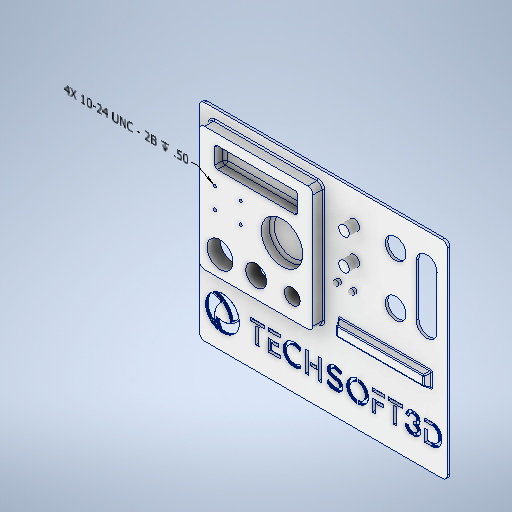
# Autodesk Inventor part: 20250213001
Saved by Autodesk Inventor 2025 (Build 290162000, 162)
## iProperties
Created: 2025-02-13
Part Number: 20250213001
Material: Aluminum 6061
Document SubType Name: Modeling
Designer: beau.trifiro
Density: 2.7 g/cm^3
Appearance: Aluminum - Flat
Description: Sample part
Mass: 1145.53 g
Surface Area: 1662.07 cm^2
Volume: 424.269 cm^3
Company: Tech Soft 3D
Author: beau.trifiro
Title: Sample Part
Revision Number: 0
Autodesk Inventor part; units mm, degrees
(part 1 of 2)
ref_plane "YZ Plane" through (0, 0, 0) normal (1, 0, 0) x (0, 1, 0)
ref_plane "XZ Plane" through (0, 0, 0) normal (0, 1, 0) x (-1, 0, 0)
ref_plane "XY Plane" through (0, 0, 0) normal (0, 0, 1) x (1, 0, 0)
sketch "Sketch1" plane through (0, 0, 0) normal (0, 0, 1) x (1, 0, 0)
  line L0 (-152.4, -127) -> (152.4, -127)
  line L1 (152.4, -127) -> (152.4, 127)
  line L2 (152.4, 127) -> (-152.4, 127)
  line L3 (-152.4, 127) -> (-152.4, -127)
  line L4 (-152.4, -127) -> (152.4, 127) construction
  line L5 (152.4, -127) -> (-152.4, 127) construction
  point P0 (0, 0)
  dimension "d0" = 304.8
  dimension "d1" = 254
  constraints: 12 end point, 2 midpoint, 2 parallel, 1 horizontal, 1 perpendicular
  measures "d0" distance of L1.end L2.end
  measures "d1" distance of L0.end L1.end
extrude "Extrusion1" add sketch "Sketch1" along normal blind 3.175
sketch "Sketch2" plane through (0, 0, 3.175) normal (0, 0, 1) x (1, 0, 0)
  line L0 (-139.7, 114.3) -> (0, 114.3)
  line L1 (0, 114.3) -> (0, -38.1)
  line L2 (0, -38.1) -> (-139.7, -38.1)
  line L3 (-139.7, -38.1) -> (-139.7, 114.3)
  line L4 (152.4, 127) -> (-152.4, 127) projected
  line L5 (-152.4, 127) -> (-152.4, -127) projected
  line L6 (-152.4, -127) -> (152.4, -127) projected
  point P0 (0, 0)
  dimension "d4" = 12.7
  dimension "d5" = 12.7
  dimension "d39" = 152.4
  constraints: 8 end point, 2 parallel, 1 horizontal, 1 perpendicular, 1 vertical alignment
  measures "d4" distance between parallel lines of L4 L0
  measures "d5" distance between parallel lines of L5 L3
  measures "d39" distance of L2.end L0.start
extrude "Extrusion2" add sketch "Sketch2" along normal blind 12.7
sketch "Sketch3" plane through (0, 0, 15.875) normal (0, 0, 1) x (1, 0, 0)
  line L0 (-120.65, 101.6) -> (-19.05, 101.6)
  line L1 (-19.05, 101.6) -> (-19.05, 76.2)
  line L2 (-19.05, 76.2) -> (-120.65, 76.2)
  line L3 (-120.65, 76.2) -> (-120.65, 101.6)
  circle A0 centre (-114.3, -12.7) radius 15.875
  circle A1 centre (-38.1, 38.1) radius 25.4
  circle A2 centre (-25.4, -12.7) radius 9.525
  circle A3 centre (-69.85, -12.7) radius 12.7
  line L4 (-139.7, 114.3) -> (-139.7, -38.1) projected
  line L5 (0, 114.3) -> (-139.7, 114.3) projected
  line L6 (0, -38.1) -> (0, 114.3) projected
  line L7 (-139.7, -38.1) -> (0, -38.1) projected
  line L8 (-120.65, 57.15) -> (-88.9, 57.15) construction
  line L9 (-88.9, 57.15) -> (-88.9, 31.75) construction
  line L10 (-88.9, 31.75) -> (-120.65, 31.75) construction
  line L11 (-120.65, 31.75) -> (-120.65, 57.15) construction
  point P0 (0, 0)
  point P1 (0, 38.1)
  point P2 (0, 38.1)
  dimension "d9" = 19.05
  dimension "d10" = 12.7
  dimension "d11" = 19.05
  dimension "d12" = 25.4
  dimension "d13" = 50.8
  dimension "d14" = 38.1
  dimension "d16" = 31.75
  dimension "d17" = 19.05
  dimension "d19" = 25.4
  dimension "d21" = 25.4
  dimension "d22" = 25.4
  dimension "d23" = 50.8
  dimension "d40" = 44.45
  dimension "d41" = 38.1
  dimension "d42" = 25.4
  dimension "d43" = 31.75
  dimension "d44" = 19.05
  dimension "d45" = 19.05
  constraints: 16 end point, 4 centre point, 4 parallel, 3 horizontal alignment, 2 horizontal, 2 midpoint, 2 perpendicular
  measures "d9" distance between parallel lines of L4 L3
  measures "d10" distance between parallel lines of L5 L0
  measures "d11" distance between parallel lines of L6 L1
  measures "d12" distance between parallel lines of L0 L2
  measures "d13" diameter of A1
  measures "d14" distance from line of L6 A1.centre
  measures "d16" diameter of A0
  measures "d17" diameter of A2
  measures "d19" diameter of A3
  measures "d21" distance from line of L4 A0.centre
  measures "d22" distance from line of L6 A2.centre
  measures "d23" vertical distance of point (0, 38.1) A2.centre
  measures "d40" distance of A2.centre A3.centre
  measures "d42" distance of L8.end L9.end
  measures "d43" distance of L9.end L10.end
  measures "d44" distance between parallel lines of L4 L11
  measures "d45" distance between parallel lines of L2 L8
extrude "Extrusion3" cut sketch "Sketch3" against normal blind 12.7 contours L0 L1 L2 L3
extrude "Extrusion4" cut sketch "Sketch3" against normal blind 12.7 contours A1
extrude "Extrusion5" cut sketch "Sketch3" against normal through all contours A0 | A2 | A3
sketch "Sketch4" plane through (0, 0, 3.175) normal (0, 0, 1) x (1, 0, 0)
  line L0 (127, 88.9) -> (127, 25.4) construction
  line L1 (114.3, 88.9) -> (114.3, 25.4)
  line L2 (139.7, 25.4) -> (139.7, 88.9)
  arc A0 (139.7, 88.9) -> (114.3, 88.9) centre (127, 88.9) ccw
  arc A1 (114.3, 25.4) -> (139.7, 25.4) centre (127, 25.4) ccw
  circle A2 centre (88.9, 88.9) radius 12.7
  circle A3 centre (88.9, 25.4) radius 12.7
  line L3 (152.4, 127) -> (-152.4, 127) projected
  line L4 (152.4, -127) -> (152.4, 127) projected
  circle A4 centre (38.1, 88.9) radius 6.35
  circle A5 centre (38.1, 50.8) radius 6.35
  circle A6 centre (38.1, 19.05) radius 3.175
  line L5 (0, -38.1) -> (0, 114.3) projected
  circle A7 centre (19.05, 19.05) radius 3.175
  line L6 (19.05, -19.05) -> (133.35, -19.05)
  line L7 (133.35, -19.05) -> (133.35, -38.1)
  line L8 (133.35, -38.1) -> (19.05, -38.1)
  line L9 (19.05, -38.1) -> (19.05, -19.05)
  line L10 (-152.4, -127) -> (152.4, -127) projected
  point P0 (0, 0)
  point P1 (127, 57.15)
  point P2 (127, 101.6)
  point P3 (139.7, 57.15)
  point P4 (114.3, 57.15)
  dimension "d55" = 25.4
  dimension "d56" = 25.4
  dimension "d57" = 63.5
  dimension "d58" = 25.4
  dimension "d59" = 25.4
  dimension "d60" = 12.7
  dimension "d61" = 12.7
  dimension "d62" = 12.7
  dimension "d63" = 38.1
  dimension "d64" = 38.1
  dimension "d65" = 6.35
  dimension "d66" = 6.35
  dimension "d67" = 19.05
  dimension "d68" = 19.05
  dimension "d70" = 38.1
  dimension "d71" = 38.1
  dimension "d72" = 107.95
  dimension "d77" = 114.3
  dimension "d78" = 19.05
  dimension "d79" = 88.9
  dimension "d80" = 19.05
  constraints: 16 end point, 8 centre point, 5 point on circle, 4 tangent, 3 horizontal alignment, 3 midpoint, 3 parallel, 3 vertical alignment, 1 horizontal, 1 perpendicular, 1 vertical
  measures "d55" distance from line of L3 point (127, 101.6)
  measures "d56" distance of point (139.7, 57.15) point (114.3, 57.15)
  measures "d57" distance of L0.start L0.end
  measures "d58" diameter of A3
  measures "d59" diameter of A2
  measures "d60" distance between parallel lines of L4 L2
  measures "d61" diameter of A4
  measures "d62" diameter of A5
  measures "d63" distance of A5.centre A4.centre
  measures "d64" distance from line of L5 A4.centre
  measures "d65" diameter of A6
  measures "d66" diameter of A7
  measures "d67" distance of A6.centre A7.centre
  measures "d68" distance from line of L5 A7.centre
  measures "d70" distance from line of L0 A3.centre
  measures "d71" distance from line of L3 A4.centre
  measures "d72" distance from line of L3 A6.centre
  measures "d77" distance of L6.start L6.end
  measures "d78" distance between parallel lines of L4 L7
  measures "d79" distance between parallel lines of L10 L8
  measures "d80" distance of L6.end L7.end
extrude "Extrusion6" cut sketch "Sketch4" against normal through all contours A0 L2 A1 L1 | A2 | A3
hole "Hole1" at (-120.65, 57.15, 15.875) at (-88.9, 57.15, 15.875) at (-88.9, 31.75, 15.875) at (-120.65, 31.75, 15.875) direction (0, 0, -1) diameter 3.683 end through all thread size "10-24 UNC" class "2B" standard "ANSI Unified Screw Threads"
extrude "Extrusion8" add sketch "Sketch4" along normal blind 12.7 contours A4 | A5
extrude "Extrusion9" add sketch "Sketch4" along normal blind 6.35 contours A6 | A7
extrude "Extrusion10" add sketch "Sketch4" along normal blind 6.35 draft -30 contours L6 L7 L8 L9
sketch "Sketch5" plane through (0, 0, 3.175) normal (0, 0, 1) x (1, 0, 0)
  line L0 (-89.5982, -73.346) -> (-72.309, -73.346)
  line L1 (-72.309, -73.346) -> (-72.309, -76.9851)
  line L2 (-72.309, -76.9851) -> (-89.5982, -76.9851)
  line L3 (-89.5982, -76.9851) -> (-89.5982, -73.346)
  line L4 (-82.806, -99.2807) -> (-82.806, -79.0998)
  line L5 (-82.806, -79.0998) -> (-79.1012, -79.0998)
  line L6 (-79.1012, -79.0998) -> (-79.1012, -99.2813)
  line L7 (-79.1012, -99.2813) -> (-82.806, -99.2813)
  line L8 (-82.806, -99.2813) -> (-82.806, -99.2807)
  line L9 (-29.191, -93.0667) -> (-27.6081, -96.5408)
  line L10 (-27.6081, -96.5408) -> (-28.0244, -96.9058)
  line L11 (-28.0244, -96.9058) -> (-28.4615, -97.248)
  line L12 (-28.4615, -97.248) -> (-28.9174, -97.5673)
  line L13 (-28.9174, -97.5673) -> (-29.3903, -97.8637)
  line L14 (-29.3903, -97.8637) -> (-29.8784, -98.1371)
  line L15 (-29.8784, -98.1371) -> (-30.3797, -98.3872)
  line L16 (-30.3797, -98.3872) -> (-30.8924, -98.6141)
  line L17 (-30.8924, -98.6141) -> (-31.4147, -98.8175)
  line L18 (-31.4147, -98.8175) -> (-31.9447, -98.9974)
  line L19 (-31.9447, -98.9974) -> (-32.4805, -99.1537)
  line L20 (-32.4805, -99.1537) -> (-33.0202, -99.2863)
  line L21 (-33.0202, -99.2863) -> (-33.562, -99.395)
  line L22 (-33.562, -99.395) -> (-34.104, -99.4797)
  line L23 (-34.104, -99.4797) -> (-34.6444, -99.5404)
  line L24 (-34.6444, -99.5404) -> (-35.1813, -99.5769)
  line L25 (-35.1813, -99.5769) -> (-35.7128, -99.5891)
  line L26 (-35.7128, -99.5891) -> (-36.4069, -99.5718)
  line L27 (-36.4069, -99.5718) -> (-37.092, -99.5205)
  line L28 (-37.092, -99.5205) -> (-37.7672, -99.4361)
  line L29 (-37.7672, -99.4361) -> (-38.4318, -99.3194)
  line L30 (-38.4318, -99.3194) -> (-39.0848, -99.1712)
  line L31 (-39.0848, -99.1712) -> (-39.7253, -98.9923)
  line L32 (-39.7253, -98.9923) -> (-40.3526, -98.7836)
  line L33 (-40.3526, -98.7836) -> (-40.9657, -98.5459)
  line L34 (-40.9657, -98.5459) -> (-41.5639, -98.2801)
  line L35 (-41.5639, -98.2801) -> (-42.1462, -97.9869)
  line L36 (-42.1462, -97.9869) -> (-42.7119, -97.6673)
  line L37 (-42.7119, -97.6673) -> (-43.26, -97.322)
  line L38 (-43.26, -97.322) -> (-43.7896, -96.9519)
  line L39 (-43.7896, -96.9519) -> (-44.3001, -96.5578)
  line L40 (-44.3001, -96.5578) -> (-44.7904, -96.1405)
  line L41 (-44.7904, -96.1405) -> (-45.2597, -95.701)
  line L42 (-45.2597, -95.701) -> (-45.7072, -95.2399)
  line L43 (-45.7072, -95.2399) -> (-46.1321, -94.7582)
  line L44 (-46.1321, -94.7582) -> (-46.5334, -94.2567)
  line L45 (-46.5334, -94.2567) -> (-46.9103, -93.7362)
  line L46 (-46.9103, -93.7362) -> (-47.262, -93.1975)
  line L47 (-47.262, -93.1975) -> (-47.5876, -92.6416)
  line L48 (-47.5876, -92.6416) -> (-47.8862, -92.0691)
  line L49 (-47.8862, -92.0691) -> (-48.1571, -91.481)
  line L50 (-48.1571, -91.481) -> (-48.3992, -90.8781)
  line L51 (-48.3992, -90.8781) -> (-48.6119, -90.2613)
  line L52 (-48.6119, -90.2613) -> (-48.7942, -89.6312)
  line L53 (-48.7942, -89.6312) -> (-48.9452, -88.9889)
  line L54 (-48.9452, -88.9889) -> (-49.0642, -88.335)
  line L55 (-49.0642, -88.335) -> (-49.1503, -87.6706)
  line L56 (-49.1503, -87.6706) -> (-49.2025, -86.9963)
  line L57 (-49.2025, -86.9963) -> (-49.2201, -86.313)
  line L58 (-49.2201, -86.313) -> (-49.2025, -85.6298)
  line L59 (-49.2025, -85.6298) -> (-49.1503, -84.9555)
  line L60 (-49.1503, -84.9555) -> (-49.0642, -84.291)
  line L61 (-49.0642, -84.291) -> (-48.9452, -83.6371)
  line L62 (-48.9452, -83.6371) -> (-48.7941, -82.9948)
  line L63 (-48.7941, -82.9948) -> (-48.6118, -82.3647)
  line L64 (-48.6118, -82.3647) -> (-48.3992, -81.7478)
  line L65 (-48.3992, -81.7478) -> (-48.157, -81.1449)
  line L66 (-48.157, -81.1449) -> (-47.8861, -80.5568)
  line L67 (-47.8861, -80.5568) -> (-47.5875, -79.9843)
  line L68 (-47.5875, -79.9843) -> (-47.2619, -79.4283)
  line L69 (-47.2619, -79.4283) -> (-46.9102, -78.8897)
  line L70 (-46.9102, -78.8897) -> (-46.5332, -78.3691)
  line L71 (-46.5332, -78.3691) -> (-46.1319, -77.8676)
  line L72 (-46.1319, -77.8676) -> (-45.707, -77.3859)
  line L73 (-45.707, -77.3859) -> (-45.2595, -76.9248)
  line L74 (-45.2595, -76.9248) -> (-44.7901, -76.4852)
  line L75 (-44.7901, -76.4852) -> (-44.2998, -76.0679)
  line L76 (-44.2998, -76.0679) -> (-43.7894, -75.6738)
  line L77 (-43.7894, -75.6738) -> (-43.2597, -75.3037)
  line L78 (-43.2597, -75.3037) -> (-42.7116, -74.9583)
  line L79 (-42.7116, -74.9583) -> (-42.146, -74.6387)
  line L80 (-42.146, -74.6387) -> (-41.5636, -74.3455)
  line L81 (-41.5636, -74.3455) -> (-40.9655, -74.0796)
  line L82 (-40.9655, -74.0796) -> (-40.3523, -73.8419)
  line L83 (-40.3523, -73.8419) -> (-39.7251, -73.6332)
  line L84 (-39.7251, -73.6332) -> (-39.0846, -73.4543)
  line L85 (-39.0846, -73.4543) -> (-38.4316, -73.3061)
  line L86 (-38.4316, -73.3061) -> (-37.7671, -73.1893)
  line L87 (-37.7671, -73.1893) -> (-37.0919, -73.1049)
  line L88 (-37.0919, -73.1049) -> (-36.4068, -73.0536)
  line L89 (-36.4068, -73.0536) -> (-35.7128, -73.0364)
  line L90 (-35.7128, -73.0364) -> (-35.1812, -73.0481)
  line L91 (-35.1812, -73.0481) -> (-34.6442, -73.0834)
  line L92 (-34.6442, -73.0834) -> (-34.1038, -73.1422)
  line L93 (-34.1038, -73.1422) -> (-33.5617, -73.2245)
  line L94 (-33.5617, -73.2245) -> (-33.0198, -73.3303)
  line L95 (-33.0198, -73.3303) -> (-32.48, -73.4597)
  line L96 (-32.48, -73.4597) -> (-31.9442, -73.6126)
  line L97 (-31.9442, -73.6126) -> (-31.4143, -73.7889)
  line L98 (-31.4143, -73.7889) -> (-30.892, -73.9889)
  line L99 (-30.892, -73.9889) -> (-30.3793, -74.2123)
  line L100 (-30.3793, -74.2123) -> (-29.878, -74.4592)
  line L101 (-29.878, -74.4592) -> (-29.39, -74.7297)
  line L102 (-29.39, -74.7297) -> (-28.9171, -75.0237)
  line L103 (-28.9171, -75.0237) -> (-28.4613, -75.3412)
  line L104 (-28.4613, -75.3412) -> (-28.0243, -75.6822)
  line L105 (-28.0243, -75.6822) -> (-27.6081, -76.0467)
  line L106 (-27.6081, -76.0467) -> (-29.191, -79.5196)
  line L107 (-29.191, -79.5196) -> (-29.5272, -79.1895)
  line L108 (-29.5272, -79.1895) -> (-29.8707, -78.8795)
  line L109 (-29.8707, -78.8795) -> (-30.2223, -78.5898)
  line L110 (-30.2223, -78.5898) -> (-30.5829, -78.3204)
  line L111 (-30.5829, -78.3204) -> (-30.9535, -78.0716)
  line L112 (-30.9535, -78.0716) -> (-31.335, -77.8435)
  line L113 (-31.335, -77.8435) -> (-31.7281, -77.6364)
  line L114 (-31.7281, -77.6364) -> (-32.134, -77.4503)
  line L115 (-32.134, -77.4503) -> (-32.5533, -77.2855)
  line L116 (-32.5533, -77.2855) -> (-32.9872, -77.1421)
  line L117 (-32.9872, -77.1421) -> (-33.4364, -77.0203)
  line L118 (-33.4364, -77.0203) -> (-33.9019, -76.9203)
  line L119 (-33.9019, -76.9203) -> (-34.3846, -76.8422)
  line L120 (-34.3846, -76.8422) -> (-34.8853, -76.7862)
  line L121 (-34.8853, -76.7862) -> (-35.4051, -76.7524)
  line L122 (-35.4051, -76.7524) -> (-35.9447, -76.7412)
  line L123 (-35.9447, -76.7412) -> (-36.4374, -76.7536)
  line L124 (-36.4374, -76.7536) -> (-36.9235, -76.7906)
  line L125 (-36.9235, -76.7906) -> (-37.4027, -76.8514)
  line L126 (-37.4027, -76.8514) -> (-37.8741, -76.9356)
  line L127 (-37.8741, -76.9356) -> (-38.3373, -77.0424)
  line L128 (-38.3373, -77.0424) -> (-38.7915, -77.1714)
  line L129 (-38.7915, -77.1714) -> (-39.2363, -77.3218)
  line L130 (-39.2363, -77.3218) -> (-39.671, -77.4932)
  line L131 (-39.671, -77.4932) -> (-40.095, -77.6848)
  line L132 (-40.095, -77.6848) -> (-40.5077, -77.8962)
  line L133 (-40.5077, -77.8962) -> (-40.9086, -78.1266)
  line L134 (-40.9086, -78.1266) -> (-41.2969, -78.3755)
  line L135 (-41.2969, -78.3755) -> (-41.6722, -78.6423)
  line L136 (-41.6722, -78.6423) -> (-42.0338, -78.9264)
  line L137 (-42.0338, -78.9264) -> (-42.3811, -79.2273)
  line L138 (-42.3811, -79.2273) -> (-42.7135, -79.5441)
  line L139 (-42.7135, -79.5441) -> (-43.0304, -79.8765)
  line L140 (-43.0304, -79.8765) -> (-43.3312, -80.2238)
  line L141 (-43.3312, -80.2238) -> (-43.6153, -80.5854)
  line L142 (-43.6153, -80.5854) -> (-43.8821, -80.9606)
  line L143 (-43.8821, -80.9606) -> (-44.1311, -81.3489)
  line L144 (-44.1311, -81.3489) -> (-44.3615, -81.7497)
  line L145 (-44.3615, -81.7497) -> (-44.5729, -82.1624)
  line L146 (-44.5729, -82.1624) -> (-44.7645, -82.5864)
  line L147 (-44.7645, -82.5864) -> (-44.9359, -83.0211)
  line L148 (-44.9359, -83.0211) -> (-45.0863, -83.4658)
  line L149 (-45.0863, -83.4658) -> (-45.2153, -83.9201)
  line L150 (-45.2153, -83.9201) -> (-45.3221, -84.3832)
  line L151 (-45.3221, -84.3832) -> (-45.4063, -84.8546)
  line L152 (-45.4063, -84.8546) -> (-45.4671, -85.3336)
  line L153 (-45.4671, -85.3336) -> (-45.5041, -85.8198)
  line L154 (-45.5041, -85.8198) -> (-45.5165, -86.3124)
  line L155 (-45.5165, -86.3124) -> (-45.5041, -86.805)
  line L156 (-45.5041, -86.805) -> (-45.4671, -87.2912)
  line L157 (-45.4671, -87.2912) -> (-45.4063, -87.7703)
  line L158 (-45.4063, -87.7703) -> (-45.3221, -88.2417)
  line L159 (-45.3221, -88.2417) -> (-45.2153, -88.7048)
  line L160 (-45.2153, -88.7048) -> (-45.0863, -89.159)
  line L161 (-45.0863, -89.159) -> (-44.9359, -89.6038)
  line L162 (-44.9359, -89.6038) -> (-44.7645, -90.0385)
  line L163 (-44.7645, -90.0385) -> (-44.5729, -90.4625)
  line L164 (-44.5729, -90.4625) -> (-44.3615, -90.8752)
  line L165 (-44.3615, -90.8752) -> (-44.1311, -91.2761)
  line L166 (-44.1311, -91.2761) -> (-43.8821, -91.6644)
  line L167 (-43.8821, -91.6644) -> (-43.6153, -92.0397)
  line L168 (-43.6153, -92.0397) -> (-43.3312, -92.4013)
  line L169 (-43.3312, -92.4013) -> (-43.0304, -92.7486)
  line L170 (-43.0304, -92.7486) -> (-42.7135, -93.081)
  line L171 (-42.7135, -93.081) -> (-42.3811, -93.3979)
  line L172 (-42.3811, -93.3979) -> (-42.0338, -93.6987)
  line L173 (-42.0338, -93.6987) -> (-41.6722, -93.9829)
  line L174 (-41.6722, -93.9829) -> (-41.2969, -94.2497)
  line L175 (-41.2969, -94.2497) -> (-40.9086, -94.4987)
  line L176 (-40.9086, -94.4987) -> (-40.5077, -94.7291)
  line L177 (-40.5077, -94.7291) -> (-40.095, -94.9405)
  line L178 (-40.095, -94.9405) -> (-39.671, -95.1322)
  line L179 (-39.671, -95.1322) -> (-39.2363, -95.3035)
  line L180 (-39.2363, -95.3035) -> (-38.7915, -95.454)
  line L181 (-38.7915, -95.454) -> (-38.3373, -95.583)
  line L182 (-38.3373, -95.583) -> (-37.8741, -95.6898)
  line L183 (-37.8741, -95.6898) -> (-37.4027, -95.774)
  line L184 (-37.4027, -95.774) -> (-36.9235, -95.8349)
  line L185 (-36.9235, -95.8349) -> (-36.4374, -95.8718)
  line L186 (-36.4374, -95.8718) -> (-35.9447, -95.8843)
  line L187 (-35.9447, -95.8843) -> (-35.4051, -95.873)
  line L188 (-35.4051, -95.873) -> (-34.8853, -95.8392)
  line L189 (-34.8853, -95.8392) -> (-34.3846, -95.783)
  line L190 (-34.3846, -95.783) -> (-33.9019, -95.7046)
  line L191 (-33.9019, -95.7046) -> (-33.4364, -95.6039)
  line L192 (-33.4364, -95.6039) -> (-32.9872, -95.4813)
  line L193 (-32.9872, -95.4813) -> (-32.5533, -95.3367)
  line L194 (-32.5533, -95.3367) -> (-32.134, -95.1702)
  line L195 (-32.134, -95.1702) -> (-31.7281, -94.9821)
  line L196 (-31.7281, -94.9821) -> (-31.335, -94.7724)
  line L197 (-31.335, -94.7724) -> (-30.9535, -94.5411)
  line L198 (-30.9535, -94.5411) -> (-30.5829, -94.2885)
  line L199 (-30.5829, -94.2885) -> (-30.2223, -94.0147)
  line L200 (-30.2223, -94.0147) -> (-29.8707, -93.7197)
  line L201 (-29.8707, -93.7197) -> (-29.5272, -93.4036)
  line L202 (-29.5272, -93.4036) -> (-29.191, -93.0667)
  line L203 (-21.72, -73.346) -> (-18.0152, -73.346)
  line L204 (-18.0152, -73.346) -> (-18.0152, -99.2807)
  line L205 (-18.0152, -99.2807) -> (-21.72, -99.2807)
  line L206 (-21.72, -99.2807) -> (-21.72, -73.346)
  line L207 (-15.8457, -88.1657) -> (-15.8457, -84.4603)
  line L208 (-15.8457, -84.4603) -> (-7.8892, -84.4603)
  line L209 (-7.8892, -84.4603) -> (-7.8892, -88.1657)
  line L210 (-7.8892, -88.1657) -> (-15.8457, -88.1657)
  line L211 (-1.9601, -73.346) -> (-1.9601, -99.2807)
  line L212 (-1.9601, -99.2807) -> (-5.6655, -99.2807)
  line L213 (-5.6655, -99.2807) -> (-5.6655, -88.1663)
  line L214 (-5.6655, -88.1663) -> (-5.6655, -84.4609)
  line L215 (-5.6655, -84.4609) -> (-5.6655, -73.346)
  line L216 (-5.6655, -73.346) -> (-1.9601, -73.346)
  line L217 (23.9204, -91.6772) -> (23.9095, -92.0971)
  line L218 (23.9095, -92.0971) -> (23.8769, -92.5101)
  line L219 (23.8769, -92.5101) -> (23.8229, -92.9158)
  line L220 (23.8229, -92.9158) -> (23.7477, -93.3136)
  line L221 (23.7477, -93.3136) -> (23.6517, -93.7032)
  line L222 (23.6517, -93.7032) -> (23.535, -94.0841)
  line L223 (23.535, -94.0841) -> (23.398, -94.456)
  line L224 (23.398, -94.456) -> (23.2408, -94.8184)
  line L225 (23.2408, -94.8184) -> (23.0639, -95.1709)
  line L226 (23.0639, -95.1709) -> (22.8673, -95.5131)
  line L227 (22.8673, -95.5131) -> (22.6514, -95.8446)
  line L228 (22.6514, -95.8446) -> (22.4165, -96.1649)
  line L229 (22.4165, -96.1649) -> (22.1627, -96.4737)
  line L230 (22.1627, -96.4737) -> (21.8905, -96.7704)
  line L231 (21.8905, -96.7704) -> (21.5999, -97.0548)
  line L232 (21.5999, -97.0548) -> (21.2913, -97.3264)
  line L233 (21.2913, -97.3264) -> (20.965, -97.5848)
  line L234 (20.965, -97.5848) -> (20.6212, -97.8295)
  line L235 (20.6212, -97.8295) -> (20.2602, -98.0601)
  line L236 (20.2602, -98.0601) -> (19.8822, -98.2763)
  line L237 (19.8822, -98.2763) -> (19.4875, -98.4776)
  line L238 (19.4875, -98.4776) -> (19.0763, -98.6635)
  line L239 (19.0763, -98.6635) -> (18.649, -98.8337)
  line L240 (18.649, -98.8337) -> (18.2057, -98.9878)
  line L241 (18.2057, -98.9878) -> (17.7468, -99.1253)
  line L242 (17.7468, -99.1253) -> (17.2725, -99.2459)
  line L243 (17.2725, -99.2459) -> (16.7831, -99.349)
  line L244 (16.7831, -99.349) -> (16.2787, -99.4343)
  line L245 (16.2787, -99.4343) -> (15.7598, -99.5014)
  line L246 (15.7598, -99.5014) -> (15.2265, -99.5498)
  line L247 (15.2265, -99.5498) -> (14.6791, -99.5792)
  line L248 (14.6791, -99.5792) -> (14.1179, -99.5891)
  line L249 (14.1179, -99.5891) -> (13.5573, -99.5783)
  line L250 (13.5573, -99.5783) -> (13.0118, -99.5469)
  line L251 (13.0118, -99.5469) -> (12.4813, -99.4962)
  line L252 (12.4813, -99.4962) -> (11.9662, -99.4273)
  line L253 (11.9662, -99.4273) -> (11.4663, -99.3417)
  line L254 (11.4663, -99.3417) -> (10.982, -99.2406)
  line L255 (10.982, -99.2406) -> (10.5132, -99.1252)
  line L256 (10.5132, -99.1252) -> (10.06, -98.9969)
  line L257 (10.06, -98.9969) -> (9.6226, -98.857)
  line L258 (9.6226, -98.857) -> (9.2011, -98.7067)
  line L259 (9.2011, -98.7067) -> (8.7956, -98.5473)
  line L260 (8.7956, -98.5473) -> (8.4062, -98.3802)
  line L261 (8.4062, -98.3802) -> (8.033, -98.2065)
  line L262 (8.033, -98.2065) -> (7.6761, -98.0277)
  line L263 (7.6761, -98.0277) -> (7.0116, -97.6594)
  line L264 (7.0116, -97.6594) -> (6.4135, -97.2857)
  line L265 (6.4135, -97.2857) -> (5.8829, -96.9169)
  line L266 (5.8829, -96.9169) -> (5.4204, -96.5632)
  line L267 (5.4204, -96.5632) -> (5.0269, -96.235)
  line L268 (5.0269, -96.235) -> (4.7034, -95.9424)
  line L269 (4.7034, -95.9424) -> (4.4505, -95.6959)
  line L270 (4.4505, -95.6959) -> (4.1605, -95.382)
  line L271 (4.1605, -95.382) -> (6.0126, -92.0632)
  line L272 (6.0126, -92.0632) -> (6.4272, -92.5005)
  line L273 (6.4272, -92.5005) -> (6.8596, -92.9145)
  line L274 (6.8596, -92.9145) -> (7.309, -93.3045)
  line L275 (7.309, -93.3045) -> (7.7741, -93.6698)
  line L276 (7.7741, -93.6698) -> (8.2539, -94.0098)
  line L277 (8.2539, -94.0098) -> (8.7473, -94.3238)
  line L278 (8.7473, -94.3238) -> (9.2533, -94.6112)
  line L279 (9.2533, -94.6112) -> (9.7708, -94.8711)
  line L280 (9.7708, -94.8711) -> (10.2987, -95.103)
  line L281 (10.2987, -95.103) -> (10.8359, -95.3062)
  line L282 (10.8359, -95.3062) -> (11.3813, -95.48)
  line L283 (11.3813, -95.48) -> (11.9339, -95.6238)
  line L284 (11.9339, -95.6238) -> (12.4926, -95.7367)
  line L285 (12.4926, -95.7367) -> (13.0563, -95.8182)
  line L286 (13.0563, -95.8182) -> (13.6239, -95.8677)
  line L287 (13.6239, -95.8677) -> (14.1944, -95.8843)
  line L288 (14.1944, -95.8843) -> (14.9044, -95.8659)
  line L289 (14.9044, -95.8659) -> (15.5723, -95.8114)
  line L290 (15.5723, -95.8114) -> (16.1975, -95.7219)
  line L291 (16.1975, -95.7219) -> (16.7796, -95.5984)
  line L292 (16.7796, -95.5984) -> (17.3181, -95.4418)
  line L293 (17.3181, -95.4418) -> (17.8124, -95.2532)
  line L294 (17.8124, -95.2532) -> (18.0428, -95.1473)
  line L295 (18.0428, -95.1473) -> (18.262, -95.0337)
  line L296 (18.262, -95.0337) -> (18.4699, -94.9126)
  line L297 (18.4699, -94.9126) -> (18.6665, -94.7842)
  line L298 (18.6665, -94.7842) -> (18.8516, -94.6485)
  line L299 (18.8516, -94.6485) -> (19.0253, -94.5057)
  line L300 (19.0253, -94.5057) -> (19.1874, -94.356)
  line L301 (19.1874, -94.356) -> (19.3379, -94.1993)
  line L302 (19.3379, -94.1993) -> (19.4767, -94.036)
  line L303 (19.4767, -94.036) -> (19.6038, -93.8661)
  line L304 (19.6038, -93.8661) -> (19.7191, -93.6897)
  line L305 (19.7191, -93.6897) -> (19.8225, -93.5069)
  line L306 (19.8225, -93.5069) -> (19.914, -93.318)
  line L307 (19.914, -93.318) -> (19.9934, -93.1229)
  line L308 (19.9934, -93.1229) -> (20.0609, -92.9219)
  line L309 (20.0609, -92.9219) -> (20.1162, -92.7151)
  line L310 (20.1162, -92.7151) -> (20.1593, -92.5025)
  line L311 (20.1593, -92.5025) -> (20.1902, -92.2844)
  line L312 (20.1902, -92.2844) -> (20.2088, -92.0608)
  line L313 (20.2088, -92.0608) -> (20.215, -91.832)
  line L314 (20.215, -91.832) -> (20.2082, -91.6389)
  line L315 (20.2082, -91.6389) -> (20.1877, -91.4506)
  line L316 (20.1877, -91.4506) -> (20.1539, -91.2669)
  line L317 (20.1539, -91.2669) -> (20.1069, -91.088)
  line L318 (20.1069, -91.088) -> (20.047, -90.9137)
  line L319 (20.047, -90.9137) -> (19.9743, -90.744)
  line L320 (19.9743, -90.744) -> (19.8892, -90.5789)
  line L321 (19.8892, -90.5789) -> (19.7917, -90.4183)
  line L322 (19.7917, -90.4183) -> (19.6821, -90.2623)
  line L323 (19.6821, -90.2623) -> (19.5606, -90.1107)
  line L324 (19.5606, -90.1107) -> (19.2828, -89.8211)
  line L325 (19.2828, -89.8211) -> (18.9601, -89.549)
  line L326 (18.9601, -89.549) -> (18.594, -89.2944)
  line L327 (18.594, -89.2944) -> (18.1863, -89.057)
  line L328 (18.1863, -89.057) -> (17.7387, -88.8366)
  line L329 (17.7387, -88.8366) -> (17.2529, -88.6329)
  line L330 (17.2529, -88.6329) -> (16.7306, -88.4457)
  line L331 (16.7306, -88.4457) -> (16.1734, -88.2747)
  line L332 (16.1734, -88.2747) -> (15.5831, -88.1199)
  line L333 (15.5831, -88.1199) -> (14.9614, -87.9808)
  line L334 (14.9614, -87.9808) -> (14.31, -87.8573)
  line L335 (14.31, -87.8573) -> (13.6485, -87.7376)
  line L336 (13.6485, -87.7376) -> (13.0167, -87.61)
  line L337 (13.0167, -87.61) -> (12.414, -87.4747)
  line L338 (12.414, -87.4747) -> (11.84, -87.3317)
  line L339 (11.84, -87.3317) -> (11.294, -87.1811)
  line L340 (11.294, -87.1811) -> (10.7753, -87.023)
  line L341 (10.7753, -87.023) -> (10.2836, -86.8576)
  line L342 (10.2836, -86.8576) -> (9.8182, -86.6848)
  line L343 (9.8182, -86.6848) -> (9.3785, -86.5048)
  line L344 (9.3785, -86.5048) -> (8.9639, -86.3176)
  line L345 (8.9639, -86.3176) -> (8.5739, -86.1234)
  line L346 (8.5739, -86.1234) -> (8.2079, -85.9221)
  line L347 (8.2079, -85.9221) -> (7.8653, -85.714)
  line L348 (7.8653, -85.714) -> (7.5457, -85.4991)
  line L349 (7.5457, -85.4991) -> (7.2482, -85.2774)
  line L350 (7.2482, -85.2774) -> (6.9726, -85.0492)
  line L351 (6.9726, -85.0492) -> (6.718, -84.8143)
  line L352 (6.718, -84.8143) -> (6.484, -84.573)
  line L353 (6.484, -84.573) -> (6.27, -84.3253)
  line L354 (6.27, -84.3253) -> (6.0755, -84.0713)
  line L355 (6.0755, -84.0713) -> (5.8998, -83.8111)
  line L356 (5.8998, -83.8111) -> (5.7424, -83.5447)
  line L357 (5.7424, -83.5447) -> (5.6027, -83.2723)
  line L358 (5.6027, -83.2723) -> (5.4801, -82.994)
  line L359 (5.4801, -82.994) -> (5.3741, -82.7098)
  line L360 (5.3741, -82.7098) -> (5.2841, -82.4197)
  line L361 (5.2841, -82.4197) -> (5.2095, -82.124)
  line L362 (5.2095, -82.124) -> (5.1497, -81.8227)
  line L363 (5.1497, -81.8227) -> (5.1042, -81.5158)
  line L364 (5.1042, -81.5158) -> (5.0725, -81.2035)
  line L365 (5.0725, -81.2035) -> (5.0538, -80.8858)
  line L366 (5.0538, -80.8858) -> (5.0477, -80.5628)
  line L367 (5.0477, -80.5628) -> (5.0573, -80.1711)
  line L368 (5.0573, -80.1711) -> (5.086, -79.785)
  line L369 (5.086, -79.785) -> (5.1338, -79.405)
  line L370 (5.1338, -79.405) -> (5.2005, -79.0315)
  line L371 (5.2005, -79.0315) -> (5.2861, -78.665)
  line L372 (5.2861, -78.665) -> (5.3904, -78.306)
  line L373 (5.3904, -78.306) -> (5.5134, -77.9548)
  line L374 (5.5134, -77.9548) -> (5.6549, -77.612)
  line L375 (5.6549, -77.612) -> (5.815, -77.2779)
  line L376 (5.815, -77.2779) -> (5.9934, -76.9531)
  line L377 (5.9934, -76.9531) -> (6.1902, -76.6379)
  line L378 (6.1902, -76.6379) -> (6.4052, -76.3327)
  line L379 (6.4052, -76.3327) -> (6.6382, -76.0382)
  line L380 (6.6382, -76.0382) -> (6.8893, -75.7546)
  line L381 (6.8893, -75.7546) -> (7.1584, -75.4825)
  line L382 (7.1584, -75.4825) -> (7.4453, -75.2222)
  line L383 (7.4453, -75.2222) -> (7.7499, -74.9743)
  line L384 (7.7499, -74.9743) -> (8.0722, -74.7391)
  line L385 (8.0722, -74.7391) -> (8.4121, -74.5172)
  line L386 (8.4121, -74.5172) -> (8.7695, -74.3089)
  line L387 (8.7695, -74.3089) -> (9.1442, -74.1147)
  line L388 (9.1442, -74.1147) -> (9.5363, -73.9351)
  line L389 (9.5363, -73.9351) -> (9.9455, -73.7704)
  line L390 (9.9455, -73.7704) -> (10.3719, -73.6213)
  line L391 (10.3719, -73.6213) -> (10.8152, -73.4879)
  line L392 (10.8152, -73.4879) -> (11.2755, -73.371)
  line L393 (11.2755, -73.371) -> (11.7527, -73.2708)
  line L394 (11.7527, -73.2708) -> (12.2465, -73.1878)
  line L395 (12.2465, -73.1878) -> (12.7571, -73.1225)
  line L396 (12.7571, -73.1225) -> (13.2842, -73.0753)
  line L397 (13.2842, -73.0753) -> (13.8278, -73.0466)
  line L398 (13.8278, -73.0466) -> (14.3877, -73.037)
  line L399 (14.3877, -73.037) -> (14.9264, -73.0477)
  line L400 (14.9264, -73.0477) -> (15.2873, -73.0672)
  line L401 (15.2873, -73.0672) -> (15.7016, -73.1015)
  line L402 (15.7016, -73.1015) -> (16.1636, -73.1545)
  line L403 (16.1636, -73.1545) -> (16.6676, -73.2303)
  line L404 (16.6676, -73.2303) -> (17.2079, -73.3329)
  line L405 (17.2079, -73.3329) -> (17.7788, -73.4663)
  line L406 (17.7788, -73.4663) -> (18.3745, -73.6345)
  line L407 (18.3745, -73.6345) -> (18.9895, -73.8416)
  line L408 (18.9895, -73.8416) -> (19.6179, -74.0915)
  line L409 (19.6179, -74.0915) -> (20.2541, -74.3883)
  line L410 (20.2541, -74.3883) -> (20.5733, -74.5555)
  line L411 (20.5733, -74.5555) -> (20.8923, -74.7359)
  line L412 (20.8923, -74.7359) -> (21.2104, -74.9301)
  line L413 (21.2104, -74.9301) -> (21.5269, -75.1385)
  line L414 (21.5269, -75.1385) -> (21.841, -75.3616)
  line L415 (21.841, -75.3616) -> (22.1521, -75.6)
  line L416 (22.1521, -75.6) -> (22.4594, -75.8541)
  line L417 (22.4594, -75.8541) -> (22.7622, -76.1244)
  line L418 (22.7622, -76.1244) -> (20.9866, -79.4817)
  line L419 (20.9866, -79.4817) -> (20.7246, -79.2347)
  line L420 (20.7246, -79.2347) -> (20.4448, -78.9873)
  line L421 (20.4448, -78.9873) -> (20.1466, -78.7417)
  line L422 (20.1466, -78.7417) -> (19.8294, -78.5001)
  line L423 (19.8294, -78.5001) -> (19.4925, -78.2649)
  line L424 (19.4925, -78.2649) -> (19.1353, -78.0382)
  line L425 (19.1353, -78.0382) -> (18.7572, -77.8225)
  line L426 (18.7572, -77.8225) -> (18.3576, -77.6198)
  line L427 (18.3576, -77.6198) -> (17.9358, -77.4325)
  line L428 (17.9358, -77.4325) -> (17.4913, -77.2628)
  line L429 (17.4913, -77.2628) -> (17.0233, -77.113)
  line L430 (17.0233, -77.113) -> (16.5313, -76.9854)
  line L431 (16.5313, -76.9854) -> (16.0147, -76.8822)
  line L432 (16.0147, -76.8822) -> (15.4728, -76.8057)
  line L433 (15.4728, -76.8057) -> (14.9049, -76.7581)
  line L434 (14.9049, -76.7581) -> (14.3106, -76.7418)
  line L435 (14.3106, -76.7418) -> (13.6632, -76.7575)
  line L436 (13.6632, -76.7575) -> (13.0526, -76.8043)
  line L437 (13.0526, -76.8043) -> (12.4795, -76.8817)
  line L438 (12.4795, -76.8817) -> (11.9446, -76.989)
  line L439 (11.9446, -76.989) -> (11.4486, -77.1258)
  line L440 (11.4486, -77.1258) -> (10.9921, -77.2913)
  line L441 (10.9921, -77.2913) -> (10.5759, -77.4852)
  line L442 (10.5759, -77.4852) -> (10.2006, -77.7067)
  line L443 (10.2006, -77.7067) -> (10.0285, -77.8277)
  line L444 (10.0285, -77.8277) -> (9.8669, -77.9554)
  line L445 (9.8669, -77.9554) -> (9.7159, -78.0898)
  line L446 (9.7159, -78.0898) -> (9.5755, -78.2307)
  line L447 (9.5755, -78.2307) -> (9.4459, -78.3781)
  line L448 (9.4459, -78.3781) -> (9.3271, -78.5319)
  line L449 (9.3271, -78.5319) -> (9.2192, -78.6922)
  line L450 (9.2192, -78.6922) -> (9.1223, -78.8587)
  line L451 (9.1223, -78.8587) -> (9.0364, -79.0314)
  line L452 (9.0364, -79.0314) -> (8.9618, -79.2102)
  line L453 (8.9618, -79.2102) -> (8.8984, -79.3952)
  line L454 (8.8984, -79.3952) -> (8.8463, -79.5861)
  line L455 (8.8463, -79.5861) -> (8.8057, -79.783)
  line L456 (8.8057, -79.783) -> (8.7765, -79.9858)
  line L457 (8.7765, -79.9858) -> (8.759, -80.1943)
  line L458 (8.759, -80.1943) -> (8.7531, -80.4086)
  line L459 (8.7531, -80.4086) -> (8.7741, -80.7724)
  line L460 (8.7741, -80.7724) -> (8.8004, -80.9452)
  line L461 (8.8004, -80.9452) -> (8.8374, -81.1122)
  line L462 (8.8374, -81.1122) -> (8.8852, -81.2736)
  line L463 (8.8852, -81.2736) -> (8.9439, -81.4296)
  line L464 (8.9439, -81.4296) -> (9.0137, -81.5803)
  line L465 (9.0137, -81.5803) -> (9.0945, -81.7259)
  line L466 (9.0945, -81.7259) -> (9.1865, -81.8666)
  line L467 (9.1865, -81.8666) -> (9.2898, -82.0025)
  line L468 (9.2898, -82.0025) -> (9.5306, -82.2609)
  line L469 (9.5306, -82.2609) -> (9.8178, -82.5024)
  line L470 (9.8178, -82.5024) -> (10.1522, -82.7285)
  line L471 (10.1522, -82.7285) -> (10.5345, -82.9406)
  line L472 (10.5345, -82.9406) -> (10.9655, -83.1401)
  line L473 (10.9655, -83.1401) -> (11.446, -83.3284)
  line L474 (11.446, -83.3284) -> (11.9769, -83.5069)
  line L475 (11.9769, -83.5069) -> (12.5588, -83.677)
  line L476 (12.5588, -83.677) -> (13.1926, -83.8402)
  line L477 (13.1926, -83.8402) -> (13.8791, -83.9978)
  line L478 (13.8791, -83.9978) -> (14.619, -84.1513)
  line L479 (14.619, -84.1513) -> (15.741, -84.3852)
  line L480 (15.741, -84.3852) -> (16.7915, -84.6395)
  line L481 (16.7915, -84.6395) -> (17.7703, -84.9166)
  line L482 (17.7703, -84.9166) -> (18.2328, -85.0645)
  line L483 (18.2328, -85.0645) -> (18.6774, -85.2189)
  line L484 (18.6774, -85.2189) -> (19.1039, -85.3803)
  line L485 (19.1039, -85.3803) -> (19.5125, -85.5488)
  line L486 (19.5125, -85.5488) -> (19.903, -85.7249)
  line L487 (19.903, -85.7249) -> (20.2756, -85.9087)
  line L488 (20.2756, -85.9087) -> (20.6301, -86.1006)
  line L489 (20.6301, -86.1006) -> (20.9665, -86.3009)
  line L490 (20.9665, -86.3009) -> (21.2849, -86.5098)
  line L491 (21.2849, -86.5098) -> (21.5853, -86.7278)
  line L492 (21.5853, -86.7278) -> (21.8675, -86.955)
  line L493 (21.8675, -86.955) -> (22.1316, -87.1918)
  line L494 (22.1316, -87.1918) -> (22.3776, -87.4384)
  line L495 (22.3776, -87.4384) -> (22.6055, -87.6952)
  line L496 (22.6055, -87.6952) -> (22.8152, -87.9624)
  line L497 (22.8152, -87.9624) -> (23.0068, -88.2404)
  line L498 (23.0068, -88.2404) -> (23.1802, -88.5295)
  line L499 (23.1802, -88.5295) -> (23.3354, -88.8299)
  line L500 (23.3354, -88.8299) -> (23.4724, -89.1419)
  line L501 (23.4724, -89.1419) -> (23.5912, -89.4659)
  line L502 (23.5912, -89.4659) -> (23.6917, -89.8021)
  line L503 (23.6917, -89.8021) -> (23.774, -90.1509)
  line L504 (23.774, -90.1509) -> (23.838, -90.5125)
  line L505 (23.838, -90.5125) -> (23.8838, -90.8872)
  line L506 (23.8838, -90.8872) -> (23.9113, -91.2753)
  line L507 (23.9113, -91.2753) -> (23.9204, -91.6772)
  line L508 (41.0169, -73.0827) -> (41.0169, -76.8002)
  line L509 (41.0169, -76.8002) -> (40.5684, -76.859)
  line L510 (40.5684, -76.859) -> (40.127, -76.9379)
  line L511 (40.127, -76.9379) -> (39.6932, -77.0364)
  line L512 (39.6932, -77.0364) -> (39.2673, -77.154)
  line L513 (39.2673, -77.154) -> (38.8499, -77.2904)
  line L514 (38.8499, -77.2904) -> (38.4414, -77.4449)
  line L515 (38.4414, -77.4449) -> (38.0424, -77.6171)
  line L516 (38.0424, -77.6171) -> (37.6533, -77.8067)
  line L517 (37.6533, -77.8067) -> (37.2745, -78.013)
  line L518 (37.2745, -78.013) -> (36.9065, -78.2356)
  line L519 (36.9065, -78.2356) -> (36.5498, -78.4741)
  line L520 (36.5498, -78.4741) -> (36.2049, -78.728)
  line L521 (36.2049, -78.728) -> (35.8723, -78.9968)
  line L522 (35.8723, -78.9968) -> (35.5523, -79.28)
  line L523 (35.5523, -79.28) -> (35.2455, -79.5772)
  line L524 (35.2455, -79.5772) -> (34.9524, -79.8879)
  line L525 (34.9524, -79.8879) -> (34.6734, -80.2117)
  line L526 (34.6734, -80.2117) -> (34.409, -80.548)
  line L527 (34.409, -80.548) -> (34.1596, -80.8964)
  line L528 (34.1596, -80.8964) -> (33.9258, -81.2564)
  line L529 (33.9258, -81.2564) -> (33.708, -81.6276)
  line L530 (33.708, -81.6276) -> (33.5067, -82.0095)
  line L531 (33.5067, -82.0095) -> (33.3223, -82.4016)
  line L532 (33.3223, -82.4016) -> (33.1553, -82.8035)
  line L533 (33.1553, -82.8035) -> (33.0062, -83.2146)
  line L534 (33.0062, -83.2146) -> (32.8754, -83.6346)
  line L535 (32.8754, -83.6346) -> (32.7635, -84.0629)
  line L536 (32.7635, -84.0629) -> (32.6708, -84.4991)
  line L537 (32.6708, -84.4991) -> (32.598, -84.9426)
  line L538 (32.598, -84.9426) -> (32.5454, -85.3931)
  line L539 (32.5454, -85.3931) -> (32.5134, -85.8501)
  line L540 (32.5134, -85.8501) -> (32.5027, -86.313)
  line L541 (32.5027, -86.313) -> (32.5134, -86.776)
  line L542 (32.5134, -86.776) -> (32.5454, -87.2329)
  line L543 (32.5454, -87.2329) -> (32.598, -87.6834)
  line L544 (32.598, -87.6834) -> (32.6709, -88.127)
  line L545 (32.6709, -88.127) -> (32.7635, -88.5632)
  line L546 (32.7635, -88.5632) -> (32.8755, -88.9915)
  line L547 (32.8755, -88.9915) -> (33.0062, -89.4115)
  line L548 (33.0062, -89.4115) -> (33.1554, -89.8226)
  line L549 (33.1554, -89.8226) -> (33.3224, -90.2245)
  line L550 (33.3224, -90.2245) -> (33.5068, -90.6167)
  line L551 (33.5068, -90.6167) -> (33.7081, -90.9986)
  line L552 (33.7081, -90.9986) -> (33.926, -91.3698)
  line L553 (33.926, -91.3698) -> (34.1598, -91.7299)
  line L554 (34.1598, -91.7299) -> (34.4092, -92.0784)
  line L555 (34.4092, -92.0784) -> (34.6736, -92.4147)
  line L556 (34.6736, -92.4147) -> (34.9526, -92.7385)
  line L557 (34.9526, -92.7385) -> (35.2458, -93.0493)
  line L558 (35.2458, -93.0493) -> (35.5526, -93.3465)
  line L559 (35.5526, -93.3465) -> (35.8725, -93.6298)
  line L560 (35.8725, -93.6298) -> (36.2052, -93.8986)
  line L561 (36.2052, -93.8986) -> (36.5501, -94.1526)
  line L562 (36.5501, -94.1526) -> (36.9068, -94.3911)
  line L563 (36.9068, -94.3911) -> (37.2747, -94.6138)
  line L564 (37.2747, -94.6138) -> (37.6535, -94.8201)
  line L565 (37.6535, -94.8201) -> (38.0426, -95.0097)
  line L566 (38.0426, -95.0097) -> (38.4417, -95.182)
  line L567 (38.4417, -95.182) -> (38.8501, -95.3366)
  line L568 (38.8501, -95.3366) -> (39.2675, -95.473)
  line L569 (39.2675, -95.473) -> (39.6933, -95.5907)
  line L570 (39.6933, -95.5907) -> (40.1271, -95.6892)
  line L571 (40.1271, -95.6892) -> (40.5685, -95.7682)
  line L572 (40.5685, -95.7682) -> (41.0169, -95.8271)
  line L573 (41.0169, -95.8271) -> (41.0169, -99.5439)
  line L574 (41.0169, -99.5439) -> (40.3802, -99.4783)
  line L575 (40.3802, -99.4783) -> (39.7528, -99.3831)
  line L576 (39.7528, -99.3831) -> (39.1354, -99.259)
  line L577 (39.1354, -99.259) -> (38.5286, -99.1068)
  line L578 (38.5286, -99.1068) -> (37.9333, -98.9271)
  line L579 (37.9333, -98.9271) -> (37.3501, -98.7206)
  line L580 (37.3501, -98.7206) -> (36.7797, -98.4881)
  line L581 (36.7797, -98.4881) -> (36.2229, -98.2303)
  line L582 (36.2229, -98.2303) -> (35.6804, -97.9479)
  line L583 (35.6804, -97.9479) -> (35.1529, -97.6416)
  line L584 (35.1529, -97.6416) -> (34.6411, -97.3122)
  line L585 (34.6411, -97.3122) -> (34.1458, -96.9603)
  line L586 (34.1458, -96.9603) -> (33.6676, -96.5867)
  line L587 (33.6676, -96.5867) -> (33.2073, -96.1921)
  line L588 (33.2073, -96.1921) -> (32.7655, -95.7772)
  line L589 (32.7655, -95.7772) -> (32.3432, -95.3427)
  line L590 (32.3432, -95.3427) -> (31.9408, -94.8894)
  line L591 (31.9408, -94.8894) -> (31.5592, -94.4179)
  line L592 (31.5592, -94.4179) -> (31.199, -93.929)
  line L593 (31.199, -93.929) -> (30.8611, -93.4233)
  line L594 (30.8611, -93.4233) -> (30.546, -92.9017)
  line L595 (30.546, -92.9017) -> (30.2546, -92.3648)
  line L596 (30.2546, -92.3648) -> (29.9875, -91.8133)
  line L597 (29.9875, -91.8133) -> (29.7455, -91.248)
  line L598 (29.7455, -91.248) -> (29.5293, -90.6696)
  line L599 (29.5293, -90.6696) -> (29.3396, -90.0787)
  line L600 (29.3396, -90.0787) -> (29.177, -89.4762)
  line L601 (29.177, -89.4762) -> (29.0425, -88.8626)
  line L602 (29.0425, -88.8626) -> (28.9365, -88.2388)
  line L603 (28.9365, -88.2388) -> (28.86, -87.6055)
  line L604 (28.86, -87.6055) -> (28.8135, -86.9633)
  line L605 (28.8135, -86.9633) -> (28.7979, -86.313)
  line L606 (28.7979, -86.313) -> (28.8135, -85.6628)
  line L607 (28.8135, -85.6628) -> (28.86, -85.0208)
  line L608 (28.86, -85.0208) -> (28.9365, -84.3875)
  line L609 (28.9365, -84.3875) -> (29.0425, -83.7638)
  line L610 (29.0425, -83.7638) -> (29.177, -83.1503)
  line L611 (29.177, -83.1503) -> (29.3396, -82.5478)
  line L612 (29.3396, -82.5478) -> (29.5293, -81.957)
  line L613 (29.5293, -81.957) -> (29.7455, -81.3786)
  line L614 (29.7455, -81.3786) -> (29.9875, -80.8134)
  line L615 (29.9875, -80.8134) -> (30.2546, -80.2619)
  line L616 (30.2546, -80.2619) -> (30.546, -79.725)
  line L617 (30.546, -79.725) -> (30.8611, -79.2034)
  line L618 (30.8611, -79.2034) -> (31.199, -78.6978)
  line L619 (31.199, -78.6978) -> (31.5592, -78.2089)
  line L620 (31.5592, -78.2089) -> (31.9408, -77.7374)
  line L621 (31.9408, -77.7374) -> (32.3432, -77.2841)
  line L622 (32.3432, -77.2841) -> (32.7655, -76.8496)
  line L623 (32.7655, -76.8496) -> (33.2073, -76.4347)
  line L624 (33.2073, -76.4347) -> (33.6676, -76.04)
  line L625 (33.6676, -76.04) -> (34.1458, -75.6664)
  line L626 (34.1458, -75.6664) -> (34.6411, -75.3145)
  line L627 (34.6411, -75.3145) -> (35.1529, -74.9851)
  line L628 (35.1529, -74.9851) -> (35.6804, -74.6788)
  line L629 (35.6804, -74.6788) -> (36.2229, -74.3964)
  line L630 (36.2229, -74.3964) -> (36.7797, -74.1386)
  line L631 (36.7797, -74.1386) -> (37.3501, -73.9061)
  line L632 (37.3501, -73.9061) -> (37.9333, -73.6996)
  line L633 (37.9333, -73.6996) -> (38.5286, -73.5199)
  line L634 (38.5286, -73.5199) -> (39.1354, -73.3676)
  line L635 (39.1354, -73.3676) -> (39.7528, -73.2435)
  line L636 (39.7528, -73.2435) -> (40.3802, -73.1483)
  line L637 (40.3802, -73.1483) -> (41.0169, -73.0827)
  line L638 (55.3494, -86.313) -> (55.3337, -86.9633)
  line L639 (55.3337, -86.9633) -> (55.2873, -87.6054)
  line L640 (55.2873, -87.6054) -> (55.2107, -88.2387)
  line L641 (55.2107, -88.2387) -> (55.1048, -88.8624)
  line L642 (55.1048, -88.8624) -> (54.9702, -89.476)
  line L643 (54.9702, -89.476) -> (54.8077, -90.0785)
  line L644 (54.8077, -90.0785) -> (54.618, -90.6693)
  line L645 (54.618, -90.6693) -> (54.4018, -91.2478)
  line L646 (54.4018, -91.2478) -> (54.1598, -91.8131)
  line L647 (54.1598, -91.8131) -> (53.8927, -92.3645)
  line L648 (53.8927, -92.3645) -> (53.6013, -92.9014)
  line L649 (53.6013, -92.9014) -> (53.2862, -93.4231)
  line L650 (53.2862, -93.4231) -> (52.9483, -93.9287)
  line L651 (52.9483, -93.9287) -> (52.5882, -94.4176)
  line L652 (52.5882, -94.4176) -> (52.2066, -94.8891)
  line L653 (52.2066, -94.8891) -> (51.8042, -95.3425)
  line L654 (51.8042, -95.3425) -> (51.3818, -95.777)
  line L655 (51.3818, -95.777) -> (50.9401, -96.1919)
  line L656 (50.9401, -96.1919) -> (50.4798, -96.5866)
  line L657 (50.4798, -96.5866) -> (50.0017, -96.9602)
  line L658 (50.0017, -96.9602) -> (49.5064, -97.3121)
  line L659 (49.5064, -97.3121) -> (48.9946, -97.6415)
  line L660 (48.9946, -97.6415) -> (48.4671, -97.9478)
  line L661 (48.4671, -97.9478) -> (47.9246, -98.2302)
  line L662 (47.9246, -98.2302) -> (47.3679, -98.488)
  line L663 (47.3679, -98.488) -> (46.7976, -98.7205)
  line L664 (46.7976, -98.7205) -> (46.2144, -98.927)
  line L665 (46.2144, -98.927) -> (45.6191, -99.1068)
  line L666 (45.6191, -99.1068) -> (45.0124, -99.259)
  line L667 (45.0124, -99.259) -> (44.395, -99.3831)
  line L668 (44.395, -99.3831) -> (43.7676, -99.4783)
  line L669 (43.7676, -99.4783) -> (43.131, -99.5439)
  line L670 (43.131, -99.5439) -> (43.131, -95.8271)
  line L671 (43.131, -95.8271) -> (43.5794, -95.7682)
  line L672 (43.5794, -95.7682) -> (44.0208, -95.6893)
  line L673 (44.0208, -95.6893) -> (44.4546, -95.5908)
  line L674 (44.4546, -95.5908) -> (44.8804, -95.4731)
  line L675 (44.8804, -95.4731) -> (45.2978, -95.3368)
  line L676 (45.2978, -95.3368) -> (45.7062, -95.1822)
  line L677 (45.7062, -95.1822) -> (46.1052, -95.01)
  line L678 (46.1052, -95.01) -> (46.4943, -94.8204)
  line L679 (46.4943, -94.8204) -> (46.873, -94.614)
  line L680 (46.873, -94.614) -> (47.241, -94.3914)
  line L681 (47.241, -94.3914) -> (47.5976, -94.1528)
  line L682 (47.5976, -94.1528) -> (47.9425, -93.8989)
  line L683 (47.9425, -93.8989) -> (48.2751, -93.6301)
  line L684 (48.2751, -93.6301) -> (48.5951, -93.3468)
  line L685 (48.5951, -93.3468) -> (48.9018, -93.0495)
  line L686 (48.9018, -93.0495) -> (49.1949, -92.7387)
  line L687 (49.1949, -92.7387) -> (49.4739, -92.4149)
  line L688 (49.4739, -92.4149) -> (49.7383, -92.0785)
  line L689 (49.7383, -92.0785) -> (49.9877, -91.7301)
  line L690 (49.9877, -91.7301) -> (50.2215, -91.37)
  line L691 (50.2215, -91.37) -> (50.4393, -90.9987)
  line L692 (50.4393, -90.9987) -> (50.6406, -90.6168)
  line L693 (50.6406, -90.6168) -> (50.825, -90.2246)
  line L694 (50.825, -90.2246) -> (50.992, -89.8227)
  line L695 (50.992, -89.8227) -> (51.1411, -89.4115)
  line L696 (51.1411, -89.4115) -> (51.2719, -88.9915)
  line L697 (51.2719, -88.9915) -> (51.3838, -88.5632)
  line L698 (51.3838, -88.5632) -> (51.4764, -88.127)
  line L699 (51.4764, -88.127) -> (51.5493, -87.6835)
  line L700 (51.5493, -87.6835) -> (51.6019, -87.2329)
  line L701 (51.6019, -87.2329) -> (51.6339, -86.776)
  line L702 (51.6339, -86.776) -> (51.6446, -86.313)
  line L703 (51.6446, -86.313) -> (51.6339, -85.8501)
  line L704 (51.6339, -85.8501) -> (51.6019, -85.3931)
  line L705 (51.6019, -85.3931) -> (51.5493, -84.9426)
  line L706 (51.5493, -84.9426) -> (51.4764, -84.4991)
  line L707 (51.4764, -84.4991) -> (51.3838, -84.0629)
  line L708 (51.3838, -84.0629) -> (51.2719, -83.6346)
  line L709 (51.2719, -83.6346) -> (51.1411, -83.2146)
  line L710 (51.1411, -83.2146) -> (50.992, -82.8035)
  line L711 (50.992, -82.8035) -> (50.825, -82.4016)
  line L712 (50.825, -82.4016) -> (50.6406, -82.0095)
  line L713 (50.6406, -82.0095) -> (50.4393, -81.6276)
  line L714 (50.4393, -81.6276) -> (50.2215, -81.2564)
  line L715 (50.2215, -81.2564) -> (49.9877, -80.8964)
  line L716 (49.9877, -80.8964) -> (49.7383, -80.548)
  line L717 (49.7383, -80.548) -> (49.4739, -80.2117)
  line L718 (49.4739, -80.2117) -> (49.1949, -79.8879)
  line L719 (49.1949, -79.8879) -> (48.9018, -79.5772)
  line L720 (48.9018, -79.5772) -> (48.5951, -79.28)
  line L721 (48.5951, -79.28) -> (48.2751, -78.9968)
  line L722 (48.2751, -78.9968) -> (47.9425, -78.728)
  line L723 (47.9425, -78.728) -> (47.5976, -78.4741)
  line L724 (47.5976, -78.4741) -> (47.241, -78.2356)
  line L725 (47.241, -78.2356) -> (46.873, -78.013)
  line L726 (46.873, -78.013) -> (46.4943, -77.8067)
  line L727 (46.4943, -77.8067) -> (46.1052, -77.6171)
  line L728 (46.1052, -77.6171) -> (45.7062, -77.4449)
  line L729 (45.7062, -77.4449) -> (45.2978, -77.2904)
  line L730 (45.2978, -77.2904) -> (44.8804, -77.154)
  line L731 (44.8804, -77.154) -> (44.4546, -77.0364)
  line L732 (44.4546, -77.0364) -> (44.0208, -76.9379)
  line L733 (44.0208, -76.9379) -> (43.5794, -76.859)
  line L734 (43.5794, -76.859) -> (43.131, -76.8002)
  line L735 (43.131, -76.8002) -> (43.131, -73.0827)
  line L736 (43.131, -73.0827) -> (43.7677, -73.1483)
  line L737 (43.7677, -73.1483) -> (44.3951, -73.2435)
  line L738 (44.3951, -73.2435) -> (45.0125, -73.3676)
  line L739 (45.0125, -73.3676) -> (45.6193, -73.5199)
  line L740 (45.6193, -73.5199) -> (46.2146, -73.6996)
  line L741 (46.2146, -73.6996) -> (46.7978, -73.906)
  line L742 (46.7978, -73.906) -> (47.3681, -74.1385)
  line L743 (47.3681, -74.1385) -> (47.9249, -74.3963)
  line L744 (47.9249, -74.3963) -> (48.4674, -74.6787)
  line L745 (48.4674, -74.6787) -> (48.9949, -74.985)
  line L746 (48.9949, -74.985) -> (49.5066, -75.3144)
  line L747 (49.5066, -75.3144) -> (50.0019, -75.6663)
  line L748 (50.0019, -75.6663) -> (50.4801, -76.0399)
  line L749 (50.4801, -76.0399) -> (50.9404, -76.4345)
  line L750 (50.9404, -76.4345) -> (51.3821, -76.8494)
  line L751 (51.3821, -76.8494) -> (51.8044, -77.2838)
  line L752 (51.8044, -77.2838) -> (52.2068, -77.7372)
  line L753 (52.2068, -77.7372) -> (52.5884, -78.2086)
  line L754 (52.5884, -78.2086) -> (52.9485, -78.6975)
  line L755 (52.9485, -78.6975) -> (53.2864, -79.2032)
  line L756 (53.2864, -79.2032) -> (53.6014, -79.7248)
  line L757 (53.6014, -79.7248) -> (53.8928, -80.2616)
  line L758 (53.8928, -80.2616) -> (54.1599, -80.8131)
  line L759 (54.1599, -80.8131) -> (54.4019, -81.3784)
  line L760 (54.4019, -81.3784) -> (54.6181, -81.9568)
  line L761 (54.6181, -81.9568) -> (54.8078, -82.5476)
  line L762 (54.8078, -82.5476) -> (54.9703, -83.1501)
  line L763 (54.9703, -83.1501) -> (55.1048, -83.7636)
  line L764 (55.1048, -83.7636) -> (55.2108, -84.3874)